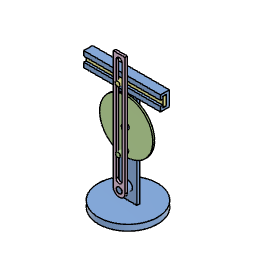
Crank and Slotted Link Mechanism v5 (Autodesk Fusion 360 design; units mm, degrees)
Autodesk Fusion 360 part; units mm, degrees
note: some values were not read from the file. Set by a fixed rule: which face or edge a step refers to.
sketch "holder stand" plane through (0, 0, 0) normal (0, 0, 1) x (1, 0, 0)
  circle A0 centre (0, 0) radius 50
  dimension "d1" = 100
  constraint coincident A0.centre origin
  measures "d1" diameter of A0
extrude "Extrude1" add sketch "holder stand" along normal blind 10 makes body 1
sketch "holder" plane through (0, 0, 10) normal (0, 0, 1) x (-1, 0, 0)
  circle A0 centre (0, 0) radius 50
  line L0 (0, 0) -> (-15, 0)
  line L1 (-15, 0) -> (-15, -5)
  line L2 (-15, -5) -> (0, -5)
  line L3 (0, -5) -> (0, 0)
  line L4 (15, -5) -> (0, -5)
  line L5 (0, 0) -> (15, 0)
  line L6 (15, 0) -> (15, -5)
  dimension "d4" = 5
  dimension "d5" = 15
  constraint horizontal L0
  constraint vertical L1
  constraint horizontal L2
  constraint vertical L3
  constraint coincident A0.centre L0.start
  constraint symmetric A0.centre L3 L0.start
  constraint symmetric L0.end L3 L5.end
  constraint symmetric L1.end L3 L4.start
  constraint symmetric L2.end L3 L4.end
  measures "d4" distance of A0.centre L2.end
  measures "d5" distance of A0.centre L0.end
extrude "Extrude2" cut sketch "holder" against normal blind 45 contours L0 L1 L2 L3 | L3 L4 L5 L6 bodies 1
extrude "Extrude3" add sketch "holder" along normal blind 190 separate body contours L0 L1 L2 L3 | L3 L4 L5 L6 makes body 2
extrude "Extrude4" add 1 faces at (5, 3.3333, 10) along direction (0, 0, -1) blind 10 on bodies 2 bodies 2
sketch "crank holder" plane through (0, 0, 0) normal (0, -1, 0) x (1, 0, 0)
  line L0 (15, 0) -> (15, 200)
  line L1 (15, 200) -> (-15, 200)
  line L2 (-15, 200) -> (-15, 0)
  line L3 (-15, 0) -> (15, 0)
  line L4 (0, 200) -> (0, 120)
  circle A0 centre (0, 120) radius 5
  dimension "d12" = 10
  constraint midpoint L1 L4.start
  constraint perpendicular L1 L4
  constraint coincident L4.end A0.centre
  measures "d12" diameter of A0
extrude "Extrude5" add sketch "crank holder" along normal blind 7 contours A0 bodies 2
sketch "crank" plane through (0, 0, 0) normal (0, -1, 0) x (1, 0, 0)
  circle A0 centre (0, 120) radius 5
  line L0 (15, 0) -> (15, 200)
  line L1 (15, 200) -> (-15, 200)
  line L2 (-15, 200) -> (-15, 0)
  line L3 (-15, 0) -> (15, 0)
  circle A1 centre (0, 120) radius 45
  dimension "d15" = 90
  constraint concentric A0 A1
  measures "d15" diameter of A1
extrude "Extrude6" add sketch "crank" along normal blind 3 separate body contours A0 | L0 L2 A1 | L0 A1 | L2 A1 makes body 3
extrude "Extrude7" cut sketch "crank" along normal blind 6 contours A0 bodies 3
move_face "OffsetFaces1" offset -0.3 1 faces at (4.9752, -4.6667, 120.4978) on bodies 2
extrude "Extrude8" add 1 faces at (-5, 3.3333, 200) along direction (0, 0, 1) blind 2 on bodies 2 bodies 2
sketch "slider holder right" plane through (15, 0, 0) normal (1, 0, 0) x (0, 1, 0)
  line L0 (5, 0) -> (5, 202)
  line L1 (5, 202) -> (0, 202)
  line L2 (0, 202) -> (0, 0)
  line L3 (0, 0) -> (5, 0)
  line L4 (0, 202) -> (5, 202)
  line L5 (5, 202) -> (5, 177)
  line L6 (5, 177) -> (0, 177)
  line L7 (0, 177) -> (0, 202)
  dimension "d23" = 25
  constraint horizontal L4
  constraint vertical L5
  constraint horizontal L6
  constraint vertical L7
  constraint coincident L1.end L2.start
  measures "d23" distance of L1.end L6.end
sketch "slider holder left" plane through (-15, 0, 0) normal (-1, 0, 0) x (0, -1, 0)
  line L0 (0, 0) -> (0, 202)
  line L1 (0, 202) -> (-5, 202)
  line L2 (-5, 202) -> (-5, 0)
  line L3 (-5, 0) -> (0, 0)
  line L4 (-5, 202) -> (0, 202)
  line L5 (0, 202) -> (0, 177)
  line L6 (0, 177) -> (-5, 177)
  line L7 (-5, 177) -> (-5, 202)
  constraint horizontal L4
  constraint vertical L5
  constraint horizontal L6
  constraint vertical L7
  constraint coincident L0 L5.end
  constraint coincident L1.end L2.start
extrude "Extrude9" add sketch "slider holder right" along normal blind 50 contours L0 L1 L2 L4 L5 L6 L7 bodies 2
extrude "Extrude10" add sketch "slider holder left" along normal blind 50 contours L0 L1 L2 L4 L5 L6 L7 bodies 2
sketch "slider holder front" plane through (0, 0, 0) normal (0, -1, 0) x (1, 0, 0)
  circle A0 centre (0, 120) radius 4.7
  line L0 (15, 0) -> (15, 177)
  line L1 (15, 177) -> (65, 177)
  line L2 (65, 177) -> (65, 202)
  line L3 (65, 202) -> (-65, 202)
  line L4 (-65, 202) -> (-65, 177)
  line L5 (-65, 177) -> (-15, 177)
  line L6 (-15, 177) -> (-15, 0)
  line L7 (-15, 0) -> (15, 0)
  line L8 (-65, 202) -> (65, 202)
  line L9 (65, 202) -> (65, 198)
  line L10 (65, 198) -> (-65, 198)
  line L11 (-65, 198) -> (-65, 202)
  line L12 (-65, 177) -> (65, 177)
  line L13 (65, 177) -> (65, 181)
  line L14 (65, 181) -> (-65, 181)
  line L15 (-65, 181) -> (-65, 177)
  dimension "d28" = 4
  dimension "d29" = 4
  constraint horizontal L8
  constraint vertical L9
  constraint horizontal L10
  constraint vertical L11
  constraint coincident L3.end L4.start
  constraint horizontal L12
  constraint vertical L13
  constraint horizontal L14
  constraint vertical L15
  constraint coincident L4.end L5.start
  constraint coincident L2 L9.end
  measures "d28" distance of L3.end L10.end
  measures "d29" distance of L4.end L14.end
extrude "Extrude11" add sketch "slider holder front" along normal blind 10 contours L1 L2 L4 L5 L12 L13 L14 L15 | L2 L3 L4 L8 L9 L10 L11 bodies 2
sketch "slider barrier bottom" plane through (0, 0, 181) normal (0, 0, 1) x (-1, 0, 0)
  line L0 (-65, 0) -> (65, 0)
  line L1 (65, 0) -> (65, 10)
  line L2 (65, 10) -> (-65, 10)
  line L3 (-65, 10) -> (-65, 0)
  line L4 (65, 10) -> (-65, 10)
  line L5 (-65, 10) -> (-65, 6)
  line L6 (-65, 6) -> (65, 6)
  line L7 (65, 6) -> (65, 10)
  dimension "d32" = 4
  constraint horizontal L4
  constraint vertical L5
  constraint horizontal L6
  constraint vertical L7
  constraint coincident L3 L5.end
  constraint coincident L1.end L2.start
  measures "d32" distance of L1.end L6.end
sketch "slider barrier top" plane through (0, 0, 198) normal (0, 0, -1) x (1, 0, 0)
  line L0 (-65, 0) -> (65, 0)
  line L1 (65, 0) -> (65, 10)
  line L2 (65, 10) -> (-65, 10)
  line L3 (-65, 10) -> (-65, 0)
  line L4 (-65, 10) -> (65, 10)
  line L5 (65, 10) -> (65, 6)
  line L6 (65, 6) -> (-65, 6)
  line L7 (-65, 6) -> (-65, 10)
  dimension "d33" = 4
  constraint horizontal L4
  constraint vertical L5
  constraint horizontal L6
  constraint vertical L7
  constraint coincident L2.end L3.start
  measures "d33" distance of L2.end L6.end
extrude "Extrude12" add sketch "slider barrier top" along normal blind 4 contours L1 L2 L3 L4 L5 L6 L7 bodies 2
extrude "Extrude13" add sketch "slider barrier bottom" along normal blind 4 contours L1 L2 L3 L4 L5 L6 L7 bodies 2
sketch "link holder" plane through (65, 0, 0) normal (1, 0, 0) x (0, 1, 0)
  line L0 (0, 177) -> (5, 177)
  line L1 (5, 177) -> (5, 202)
  line L2 (5, 202) -> (-10, 202)
  line L3 (-10, 202) -> (-10, 194)
  line L4 (-10, 194) -> (-6, 194)
  line L5 (-6, 194) -> (-6, 198)
  line L6 (-6, 198) -> (0, 198)
  line L7 (0, 198) -> (0, 181)
  line L8 (0, 181) -> (-6, 181)
  line L9 (-6, 181) -> (-6, 185)
  line L10 (-6, 185) -> (-10, 185)
  line L11 (-10, 185) -> (-10, 177)
  line L12 (-10, 177) -> (0, 177)
  line L13 (-6, 198) -> (0, 198)
  line L14 (0, 198) -> (0, 181)
  line L15 (0, 181) -> (-6, 181)
  line L16 (-6, 181) -> (-6, 198)
  constraint horizontal L13
  constraint vertical L14
  constraint horizontal L15
  constraint vertical L16
  constraint coincident L7.end L8.start
  constraint coincident L5.end L6.start
extrude "Extrude14" add sketch "link holder" against normal blind 130 separate body contours L5 L6 L7 L8 L9 L13 L14 L15 L16 makes body 4
move_face "OffsetFaces2" offset -0.3 6 faces at (21.6667, -6, 188) (-21.6667, -6, 195.3333) (-21.6667, -6, 182.3333) (21.6667, -4, 198) (-21.6667, 0, 192.3333) (21.6667, -2, 181) on bodies 4
sketch "slider" plane through (0, 0, 0) normal (0, -1, 0) x (1, 0, 0)
  circle A0 centre (0, 120) radius 4.7
  line L0 (15, 177) -> (-15, 177)
  line L1 (-15, 177) -> (-15, 0)
  line L2 (-15, 0) -> (15, 0)
  line L3 (15, 0) -> (15, 177)
  circle A1 centre (0, 32) radius 5
  dimension "d41" = 10
  measures "d41" diameter of A1
extrude "Extrude15" add sketch "slider" along normal blind 15 contours A1 bodies 2
sketch "slotted link" plane through (0, -15, 0) normal (0, -1, 0) x (1, 0, 0)
  circle A0 centre (0, 32) radius 5
  circle A1 centre (0, 32) radius 10
  line L0 (-10, 32) -> (10, 32)
  line L1 (-10, 32) -> (10, 32)
  line L2 (10, 32) -> (10, 232)
  line L3 (10, 232) -> (-10, 232)
  line L4 (-10, 232) -> (-10, 32)
  line L5 (-5, 32) -> (5, 32)
  line L6 (5, 32) -> (5, 227)
  line L7 (5, 227) -> (-5, 227)
  line L8 (-5, 227) -> (-5, 32)
  circle A2 centre (0, 222) radius 5
  circle A3 centre (0, 47) radius 5
  dimension "d44" = 5
  dimension "d45" = 20
  dimension "d46" = 200
  dimension "d47" = 195
  constraint coincident A1 L0.start
  constraint coincident A1 L0.end
  constraint horizontal L0
  constraint horizontal L1
  constraint vertical L2
  constraint horizontal L3
  constraint vertical L4
  constraint horizontal L5
  constraint vertical L6
  constraint horizontal L7
  constraint vertical L8
  constraint coincident L1 L5.start
  constraint coincident A0 L5.start
  constraint tangent L7 A2
  measures "d44" distance of A0
  measures "d45" distance of L0.start L0.end
  measures "d46" distance of L0.start L3.end
  measures "d47" distance of L5.start L7.end
extrude "Extrude16" add sketch "slotted link" against normal blind 4 separate body contours A0 A1 L0 L1 | A1 L0 L1 L6 | A0 A1 L6 L8 | A1 L0 L1 L8 | A1 L2 L3 L4 L6 L7 L8 | A1 L6 A3 | A1 L8 A3 | L6 L7 A2 | L7 L8 A2 makes body 5
move_face "OffsetFaces3" offset -0.3 1 faces at (4.9752, -10, 31.5022) on bodies 2
sketch "slotted link holder" plane through (0, -15, 0) normal (0, -1, 0) x (1, 0, 0)
  circle A0 centre (0, 32) radius 4.7
  circle A1 centre (0, 32) radius 7.5
  dimension "d52" = 15
  constraint concentric A0 A1
  measures "d52" diameter of A1
extrude "Extrude17" add sketch "slotted link holder" along normal blind -15 and the other way blind 4 bodies 2
sketch "crank pin" plane through (0, -3, 0) normal (0, -1, 0) x (1, 0, 0)
  circle A0 centre (0, 120) radius 5
  circle A1 centre (0, 120) radius 45
  circle A2 centre (0, 85) radius 4
  dimension "d57" = 8
  measures "d57" diameter of A2
sketch "slider pin" plane through (0, -5.7, 0) normal (0, -1, 0) x (1, 0, 0)
  line L0 (65, 181.3) -> (65, 197.7)
  line L1 (65, 197.7) -> (-65, 197.7)
  line L2 (-65, 197.7) -> (-65, 181.3)
  line L3 (-65, 181.3) -> (65, 181.3)
  circle A0 centre (0, 189.5) radius 4
  dimension "d58" = 8
  measures "d58" diameter of A0
extrude "Extrude18" add sketch "slider pin" along normal blind 12 contours A0 bodies 4
extrude "Extrude19" add sketch "crank pin" along normal blind 14 contours A2 bodies 3
copy_body "Body->Comp1" bodies 1 removing the originals makes body 6 in component "holder stand"
copy_body "Body->Comp2" bodies 2 removing the originals makes body 7 in component "holder"
copy_body "Body->Comp3" bodies 3 removing the originals makes body 8 in component "crank"
copy_body "Body->Comp4" bodies 4 removing the originals makes body 9 in component "slider"
copy_body "Body->Comp5" bodies 5 removing the originals makes body 10 in component "slotted link"
component "holder stand" placed x (1, 0, 0) y (0, 1, 0) z (0, 0, 1) at (0, 0, 0)
component "holder" placed x (1, 0, 0) y (0, 1, 0) z (0, 0, 1) at (0, 0, 0)
component "crank" placed x (1, 0, 0) y (0, 1, 0) z (0, 0, 1) at (0, 0, 0)
component "slider" placed x (1, 0, 0) y (0, 1, 0) z (0, 0, 1) at (0, 0, 0)
component "slotted link" placed x (1, 0, 0) y (0, 1, 0) z (0, 0, 1) at (0, 0, 0)
named bodies: "holder stand", "holder", "crank", "slider", "slotted link"
